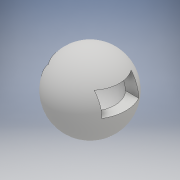
# Autodesk Inventor part: Шар
Saved by Autodesk Inventor 2018 (Build 220112000, 112)
## iProperties
Created: 2018-05-16
Part Number: Шар
Material: Типовые
Document SubType Name: Modeling
Designer: user
Density: 1 g/cm^3
Appearance: По умолчанию
Author: user
Autodesk Inventor part; units mm, degrees
ref_plane "YZ Plane" through (0, 0, 0) normal (1, 0, 0) x (0, 1, 0)
ref_plane "XZ Plane" through (0, 0, 0) normal (0, 1, 0) x (-1, 0, 0)
ref_plane "XY Plane" through (0, 0, 0) normal (0, 0, 1) x (1, 0, 0)
sketch "Эскиз1" plane through (0, 0, 0) normal (0, 0, 1) x (1, 0, 0)
  circle A0 centre (0, 0) radius 35
  line L0 (0, 35) -> (0, -35)
  dimension "d0" = 70
  constraints: 2 end point, 2 point on circle, 1 centre point, 1 coincident
  measures "d0" diameter of A0
revolve "Вращение1" add sketch "Эскиз1" angle 360 about axis through (0, 35, 0) along (0, -1, 0)
sketch "Эскиз2" plane through (0, 0, 0) normal (1, 0, 0) x (0, 1, 0)
  circle A0 centre (-0.8026, 0) radius 25
  line L0 (24.1974, 0) -> (-25.8026, 0)
  point P0 (0, 0)
  dimension "d2" = 50
  constraints: 2 end point, 2 point on circle, 1 centre point, 1 horizontal
  measures "d2" diameter of A0
revolve "Вращение2" cut sketch "Эскиз2" angle 360 about axis through (0, 24.1974, 0) along (0, -1, 0) picked at (-3.9998, -9.7861) contours A0 L0
sketch "Эскиз3" plane through (0, 0, 0) normal (1, 0, 0) x (0, 1, 0)
  circle A0 centre (-0.8026, 0) radius 25 projected
  line L0 (16.7899, 17.7624) -> (-18.4199, 17.7624)
  line L1 (-18.4199, 17.7624) -> (-18.4199, 0)
  line L2 (-18.4199, 0) -> (16.7899, 0)
  line L3 (16.7899, 0) -> (16.7899, 17.7624)
  line L4 (16.7899, 0) -> (-18.2101, 0)
  line L5 (-18.2101, 0) -> (-18.2101, 20)
  line L6 (-18.2101, 20) -> (16.7899, 20)
  line L7 (16.7899, 20) -> (16.7899, 0)
  point P0 (0, 0)
  dimension "d4" = 35
  dimension "d5" = 20
  constraints: 16 end point, 4 parallel, 2 horizontal, 2 perpendicular, 2 other
  measures "d4" distance of L5.end L6.end
  measures "d5" distance of L4.end L5.end
extrude "Выдавливание1" cut sketch "Эскиз3" along normal mid plane 100 contours L0 L5 A0 L6 | L3 L2 L5 L0 | A0 L6 L7 | A0 L5 L6
